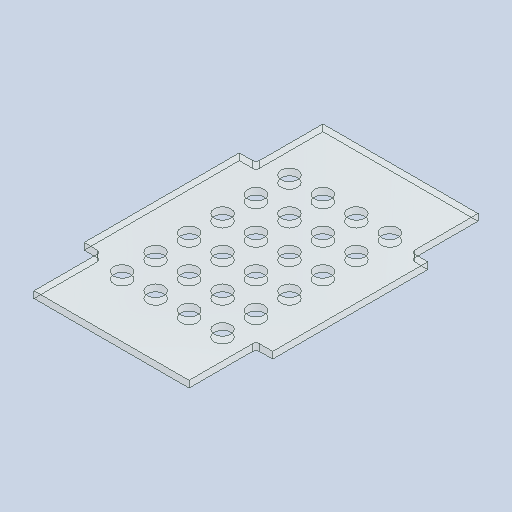
# Autodesk Inventor part: Schutzglas
Saved by Autodesk Inventor 2022 (Build 260153000, 153)
## iProperties
Created: 2021-04-25
Part Number: Schutzglas
Material: Glas
Document SubType Name: Modeling
Designer: Sebastian Seewald
Mass: 394.504 g
Surface Area: 938.858 cm^2
Volume: 180.965 cm^3
Density: 2.18 g/cm^3
Appearance: Klar
Author: Sebastian Seewald
Autodesk Inventor part; units mm, degrees
ref_plane "YZ Plane" through (0, 0, 0) normal (1, 0, 0) x (0, 1, 0)
ref_plane "XZ Plane" through (0, 0, 0) normal (0, 1, 0) x (-1, 0, 0)
ref_plane "XY Plane" through (0, 0, 0) normal (0, 0, 1) x (1, 0, 0)
sketch "Skizze1" plane through (0, 0, 0) normal (0, 0, 1) x (1, 0, 0)
  line L0 (-56.35, 2) -> (56.35, 2)
  line L1 (56.35, 2) -> (56.35, -2)
  line L2 (56.35, -2) -> (-56.35, -2)
  line L3 (-56.35, -2) -> (-56.35, 2)
  line L4 (-56.35, 2) -> (56.35, -2) construction
  line L5 (56.35, 2) -> (-56.35, -2) construction
  point P0 (0, 0)
  dimension "d0" = 4
  dimension "d1" = 112.7
  constraints: 12 end point, 2 midpoint, 2 parallel, 1 horizontal, 1 perpendicular
  measures "d0" distance of L2.end L0.start
  measures "d1" distance between parallel lines of L3 L1
extrude "Extrusion1" add sketch "Skizze1" along normal blind 172.7
sketch "Skizze2" plane through (-56.35, 2, 0) normal (0, 1, 0) x (1, 0, 0)
  circle A0 centre (26.35, -36.35) radius 5
  line L0 (112.7, 0) -> (0, 0) projected
  line L1 (0, 0) -> (0, -172.7) projected
  point P0 (56.35, 0)
  dimension "d4" = 10
  dimension "d5" = 36.35
  dimension "d6" = 26.35
  constraints: 1 centre point
  measures "d4" diameter of A0
  measures "d5" distance from line of L0 A0.centre
  measures "d6" distance from line of A0.centre L1
extrude "Extrusion2" cut sketch "Skizze2" against normal blind 10
pattern_linear "Rechteckige Anordnung1" count 4 spacing 20 along (1, 0, 0) count 6 spacing 20 along (0, 0, 1) of "Extrusion2"
sketch "Skizze3" plane through (-56.35, 2, 0) normal (0, 1, 0) x (1, 0, 0)
  line L0 (0, -172.7) -> (112.7, -172.7) projected
  line L1 (0, -172.7) -> (0, -132.7)
  line L2 (0, 0) -> (0, -172.7) projected
  line L3 (0, -172.7) -> (10, -172.7)
  line L4 (0, 0) -> (112.7, 0) projected
  line L5 (0, 0) -> (0, -40)
  line L6 (0, 0) -> (10, 0)
  line L7 (112.7, -172.7) -> (102.7, -172.7)
  line L8 (112.7, 0) -> (112.7, -172.7) projected
  line L9 (112.7, -172.7) -> (112.7, -132.7)
  line L10 (112.7, 0) -> (102.7, 0)
  line L11 (112.7, 0) -> (112.7, -40)
  line L12 (10, -172.7) -> (10, -132.7)
  line L13 (10, -132.7) -> (0, -132.7)
  line L14 (10, 0) -> (10, -40)
  line L15 (10, -40) -> (0, -40)
  circle A0 centre (106.35, -176.35) radius 5 projected
  line L16 (102.7, -172.7) -> (102.7, -132.7)
  line L17 (102.7, -132.7) -> (112.7, -132.7)
  line L18 (102.7, 0) -> (102.7, -40)
  line L19 (102.7, -40) -> (112.7, -40)
  point P0 (56.35, 0)
  point P1 (10, 0)
  point P2 (112.7, -172.9328)
  point P3 (112.7, -179.7672)
  dimension "d15" = 40
  dimension "d17" = 40
  dimension "d19" = 40
  dimension "d20" = 10
  dimension "d21" = 40
  dimension "d22" = 10
  dimension "d25" = 10
  dimension "d26" = 10
  constraints: 32 end point, 7 point on line, 4 perpendicular, 3 vertical, 2 horizontal, 1 other
  measures "d15" distance of L0.start L1.end
  measures "d17" distance from line of L4 L5.end
  measures "d19" distance from line of L10 L11.end
  measures "d20" distance from line of L8 L10.end
  measures "d21" distance from line of L0 L9.end
  measures "d22" distance from line of L9 L7.end
  measures "d25" distance between parallel lines of L2 L14
  measures "d26" distance between parallel lines of L2 L12
extrude "Extrusion3" cut sketch "Skizze3" against normal blind 10 contours L1 L13 L12 L0 | L16 L17 L8 L0 A0 | L2 L4 L14 L15 | A0 L0 | L19 L18 L4 L8 picked at (107.164, -172.1209)
fillet "Rundung1" radius 2 4 edges at (-46.35, 0, 132.7) (-46.35, 0, 40) (46.35, 0, 40) (46.35, 0, 132.7)
